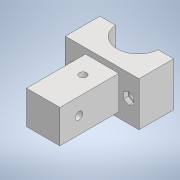
# Autodesk Inventor part: 2_Connettore_inf_sup
Saved by Autodesk Inventor 2020 (Build 240168000, 168)
## iProperties
Created: 2019-10-11
Part Number: 2_Connettore_inf_sup
Material: Generico
Document SubType Name: Modeling
Designer: socci
Density: 1 g/cm^3
Appearance: Default
Author: socci
Autodesk Inventor part; units mm, degrees
ref_plane "YZ Plane" through (0, 0, 0) normal (1, 0, 0) x (0, 1, 0)
ref_plane "XZ Plane" through (0, 0, 0) normal (0, 1, 0) x (-1, 0, 0)
ref_plane "XY Plane" through (0, 0, 0) normal (0, 0, 1) x (1, 0, 0)
sketch "Schizzo1" plane through (0, 0, 0) normal (0, 0, 1) x (1, 0, 0)
  line L0 (11.3, -11.3) -> (-11.3, -11.3)
  line L1 (-11.3, -11.3) -> (-11.3, 11.3)
  line L2 (-11.3, 11.3) -> (11.3, 11.3)
  line L3 (11.3, 11.3) -> (11.3, -11.3)
  point P0 (0, 0)
  point P1 (0, 0)
  dimension "d0" = 22.6
  constraints: 8 end point, 1 coincident, 9 other
  measures "d0" distance of L1.end L2.end
extrude "Estrusione1" add sketch "Schizzo1" along normal blind 40
sketch "Schizzo2" plane through (0, 0, 0) normal (0, 0, -1) x (-1, 0, 0)
  line L0 (25, -15) -> (-25, -15)
  line L1 (-25, -15) -> (-25, 15)
  line L2 (-25, 15) -> (25, 15)
  line L3 (25, 15) -> (25, -15)
  line L4 (25, -15) -> (-25, 15) construction
  line L5 (-25, -15) -> (25, 15) construction
  point P0 (0, 0)
  dimension "d3" = 50
  dimension "d4" = 30
  constraints: 12 end point, 3 midpoint, 2 parallel, 1 horizontal, 1 perpendicular
  measures "d3" distance of L0.start L0.end
  measures "d4" distance of L0.end L1.end
extrude "Estrusione2" add sketch "Schizzo2" along normal blind 23.5
sketch "Schizzo3" plane through (-25, 15, 0) normal (0, 1, 0) x (1, 0, 0)
  circle A0 centre (25, 24.6032) radius 14.5
  point P0 (25, 0)
  dimension "d7" = 29
  constraints: 1 centre point
  measures "d7" diameter of A0
extrude "Estrusione3" cut sketch "Schizzo3" against normal blind 30
sketch "Schizzo4" plane through (0, 0, 0) normal (0, 0, 1) x (1, 0, 0)
  line L0 (-25, -15) -> (-25, 15) projected
  line L1 (-25, 0) -> (-18, 0)
  line L2 (0, 0) -> (-18, 0)
  line L3 (-14.458, 15) -> (-14.458, -15) projected
  line L4 (0, 0) -> (18, 0)
  dimension "d14" = 18
  dimension "d15" = 18
  constraints: 6 end point, 2 horizontal, 1 midpoint, 1 perpendicular
  measures "d14" distance of L2.start L1.end
  measures "d15" distance of L2.start L4.end
hole "Foro1" at (-18, 0, 0) at (18, 0, 0) direction (0, 0, -1) diameter 5 end through all
sketch "Schizzo5" plane through (0, 0, 0) normal (0, 0, 1) x (1, 0, 0)
  circle A0 centre (-18, 0) radius 2.5 projected
  circle A1 centre (18, 0) radius 2.5 projected
  line L0 (-14.5, -2.0207) -> (-18, -4.0415)
  line L1 (-18, -4.0415) -> (-21.5, -2.0207)
  line L2 (-21.5, -2.0207) -> (-21.5, 2.0207)
  line L3 (-21.5, 2.0207) -> (-18, 4.0415)
  line L4 (-18, 4.0415) -> (-14.5, 2.0207)
  line L5 (-14.5, 2.0207) -> (-14.5, -2.0207)
  line L6 (21.5, -2.0207) -> (18, -4.0415)
  line L7 (18, -4.0415) -> (14.5, -2.0207)
  line L8 (14.5, -2.0207) -> (14.5, 2.0207)
  line L9 (14.5, 2.0207) -> (18, 4.0415)
  line L10 (18, 4.0415) -> (21.5, 2.0207)
  line L11 (21.5, 2.0207) -> (21.5, -2.0207)
  point P0 (0, 0)
  point P1 (-14.5, 0)
  point P2 (21.5, 0)
  constraints: 24 end point, 2 coincident, 2 midpoint, 26 other
extrude "Estrusione4" cut sketch "Schizzo5" against normal blind 3.2 contours A0 | A1 | L0 L1 L2 L3 L4 L5 | L6 L7 L8 L9 L10 L11
sketch "Schizzo6" plane through (-11.3, 11.3, 40) normal (0, 1, 0) x (1, 0, 0)
  line L0 (11.3, 40) -> (11.3, 27)
  line L1 (0, 0) -> (22.6, 0) projected
  line L2 (11.3, 40) -> (24.3, 40) construction
  dimension "d27" = 13
  dimension "d28" = 90
  constraints: 4 end point, 2 perpendicular, 1 horizontal
  measures "d27" distance of L0.start L0.end
  measures "d28" angle of L0 L2
hole "Foro2" at (0, 11.3, 13) direction (0, -1, 0) diameter 5 end through all
sketch "Schizzo7" plane through (-11.3, -11.3, 40) normal (-1, 0, 0) x (0, 0, 1)
  line L0 (0, 0) -> (0, 22.6) projected
  line L1 (0, 11.3) -> (-13, 11.3)
  point P0 (-40, 11.3)
  dimension "d36" = 13
  constraints: 2 end point, 1 horizontal, 1 midpoint
  measures "d36" distance of L1.start L1.end
hole "Foro3" at (-11.3, 0, 27) direction (1, 0, 0) diameter 5 end through all
